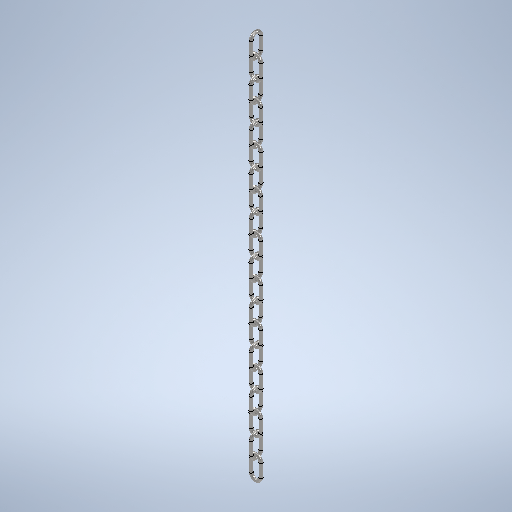
# Autodesk Inventor part: リンクチェーン
Saved by Autodesk Inventor 2025.4 (Build 294407000, 407)
## iProperties
Manager: A Shiramizu
Company: Eiko Engineering
Created: 2025-07-13
Part Number: リンクチェーン
Material: SS400
Document SubType Name: Modeling
Designer: A Shiramizu
Density: 7.98 g/cm^3
Appearance: 半つや出し
Author: huma2
Comments: 免責事項 本3Dモデルは設計検討・参考用データです。寸法、形状、強度、材質、規格適合性、使用目的への適合性は保証しません。実際の設計・製作・使用にあたっては、利用者の責任でメーカー資料、規格、法令、現物確認、強度確認等を行ってください。 本データの使用・改変・流用・再配布により生じた損害、事故、不具合等について、作成者は一切責任を負いません。 Disclaimer This 3D model and related data are provided for reference and design study purposes only. The creator makes no warranty regarding dimensions, geometry, strength, material, standards compliance, or fitness for any particular purpose. Before actual design, fabrication, installation, purchase, or use, the user must verify all information, including actual products, manufacturer data, applicable standards, laws, and strength calculations. The creator shall not be liable for any damage, accident, defect, loss, or trouble arising from the use, modification, reuse, or redistribution of this data. Use of this data is entirely at the user’s own risk.
Autodesk Inventor part; units mm, degrees
ref_plane "YZ Plane" through (0, 0, 0) normal (1, 0, 0) x (0, 1, 0)
ref_plane "XZ Plane" through (0, 0, 0) normal (0, 1, 0) x (-1, 0, 0)
sketch "スケッチ1" plane through (0, 0, 0) normal (0, 0, 1) x (1, 0, 0)
  line L0 (0, -10) -> (0, 10) construction
  line L1 (-7.5, -10) -> (-7.5, 10)
  line L2 (7.5, 10) -> (7.5, -10)
  arc A0 (-7.5, -10) -> (7.5, -10) centre (0, -10) ccw
  arc A1 (7.5, 10) -> (-7.5, 10) centre (0, 10) ccw
  point P0 (0, 0)
  dimension "d0" = 20
  dimension "d1" = 15
  constraints: 8 end point, 4 point on circle, 4 tangent, 2 centre point, 1 midpoint, 1 parallel, 1 vertical
  measures "d0" distance of L0.start L0.end
  measures "d1" distance between parallel lines of L2 L1
sketch "スケッチ2" plane through (0, 0, 0) normal (0, 1, 0) x (-1, 0, 0)
  circle A0 centre (7.5, 0) radius 2.5
  point P0 (0, 0)
  point P1 (7.5, 0)
  point P2 (7.5, 0)
  point P3 (7.5, 0)
  dimension "d2" = 5
  constraints: 1 centre point, 1 coincident
  measures "d2" diameter of A0
sweep "スイープ1" add profiles "スケッチ2" path "スケッチ1"
sketch "スケッチ3" plane through (0, 0, 0) normal (1, 0, 0) x (0, 1, 0)
  arc A0 (17.5, -2.5) -> (17.5, 2.5) centre (17.5, 0) ccw projected
  line L0 (20, 0) -> (40, 0) construction
  line L1 (20, 7.5) -> (40, 7.5)
  line L2 (40, -7.5) -> (20, -7.5)
  arc A1 (20, 7.5) -> (20, -7.5) centre (20, 0) ccw
  arc A2 (40, -7.5) -> (40, 7.5) centre (40, 0) ccw
  arc A3 (17.5, 2.5) -> (17.5, -2.5) centre (17.5, 0) ccw projected
  point P0 (0, 0)
  point P1 (30, 0)
  point P2 (12.5, 0)
  point P3 (15, 0)
  dimension "d5" = 20
  dimension "d6" = 15
  dimension "d7" = 2.5
  constraints: 8 end point, 6 point on circle, 4 tangent, 2 centre point, 1 horizontal, 1 horizontal alignment, 1 midpoint, 1 parallel
  measures "d5" distance of L0.start L0.end
  measures "d6" distance between parallel lines of L2 L1
  measures "d7" distance of point (12.5, 0) point (15, 0)
ref_plane "作業平面1" through (0, 20, 7.5) normal (0, 1, 0) x (-1, 0, 0)
sketch "スケッチ4" plane through (0, 20, 7.5) normal (0, 1, 0) x (-1, 0, 0)
  circle A0 centre (0, 0) radius 2.5
  point P0 (0, -7.5)
  dimension "d8" = 5
  constraints: 1 centre point, 1 coincident
  measures "d8" diameter of A0
sweep "スイープ2" add profiles "スケッチ4" path "スケッチ3" path curves L1 A2 L2 A1
pattern_linear "矩形状パターン1" count 10 spacing 60 along (0, 1, 0) of "スイープ1", "スイープ2"
equation "\"d0\" = -d1 + LD - DD"
equation "\"d1\" = WD"
equation "\"d2\" = DD"
equation "\"d5\" = d0"
equation "\"d6\" = d1"
equation "\"d7\" = 0.5 * d2"
equation "\"d8\" = d2"
equation "\"d13\" = 2 * d1 + 2 * d0 - 2 * d2"
equation "\"LD\" = 40"
equation "\"WD\" = 15"
equation "\"DD\" = 5"
